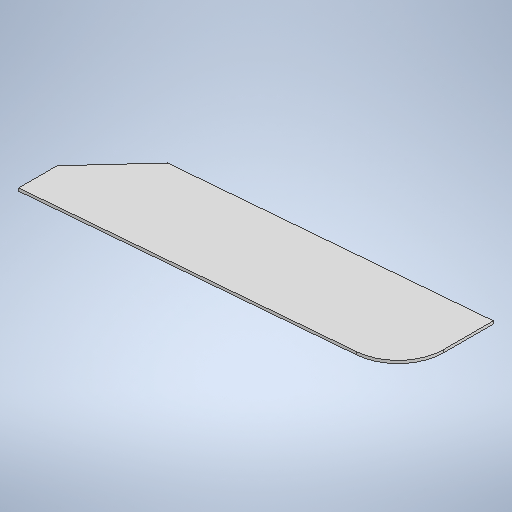
# Autodesk Inventor part: f
Saved by Autodesk Inventor 2025.2 (Build 292293000, 293)
## iProperties
Created: 2026-02-05
Part Number: f
Material: Generic
Document SubType Name: Modeling
Designer: Joefi
Density: 1 g/cm^3
Appearance: Default
Author: Joefi
Autodesk Inventor part; units mm, degrees
ref_plane "YZ Plane" through (0, 0, 0) normal (1, 0, 0) x (0, 1, 0)
ref_plane "XZ Plane" through (0, 0, 0) normal (0, 1, 0) x (-1, 0, 0)
ref_plane "XY Plane" through (0, 0, 0) normal (0, 0, 1) x (1, 0, 0)
sketch "Sketch1" plane through (0, 0, 0) normal (0, 1, 0) x (-1, 0, 0)
  line L0 (49.034, 47.4336) -> (49.034, 46.8346)
  arc A0 (47.7204, 43.4566) -> (49.034, 46.8346) centre (44.034, 46.8346) ccw
  line L1 (47.7204, 43.4566) -> (36.3172, 31.0122)
  arc A1 (33.0666, 29.4092) -> (36.3172, 31.0122) centre (32.6308, 34.3902) ccw
  line L2 (33.0666, 29.4092) -> (-42.1497, 22.8286)
  arc A2 (-47.5855, 27.8096) -> (-42.1497, 22.8286) centre (-42.5855, 27.8096) ccw
  line L3 (-47.5855, 27.8096) -> (-47.5855, 34.3574)
  arc A3 (-37.5442, 45.3156) -> (-47.5855, 34.3574) centre (-36.5855, 34.3574) ccw
  line L4 (-37.5442, 45.3156) -> (43.5982, 52.4146)
  arc A4 (49.034, 47.4336) -> (43.5982, 52.4146) centre (44.034, 47.4336) ccw
  line L5 (35.9527, 27.654) -> (51.034, 44.1124)
  line L6 (51.034, 44.1124) -> (51.034, 55.0728)
  line L7 (51.034, 55.0728) -> (-37.7185, 47.308)
  arc A5 (-37.7185, 47.308) -> (-49.5855, 34.3574) centre (-36.5855, 34.3574) ccw
  line L8 (-49.5855, 34.3574) -> (-49.5855, 20.1704)
  line L9 (-49.5855, 20.1704) -> (35.9527, 27.654)
  line L10 (35.8578, 27.8465) -> (50.834, 44.1902)
  line L11 (50.834, 44.1902) -> (50.834, 54.8545)
  line L12 (50.834, 54.8545) -> (-37.7011, 47.1087)
  arc A6 (-37.7011, 47.1087) -> (-49.3855, 34.3574) centre (-36.5855, 34.3574) ccw
  line L13 (-49.3855, 34.3574) -> (-49.3855, 20.3887)
  line L14 (-49.3855, 20.3887) -> (35.8578, 27.8465)
  dimension "d0" = 0.2
  constraints: 30 end point, 14 point on circle, 7 centre point, 5 other
  measures "d0" distance between parallel lines of L9 L14
extrude "Extrusion1" add sketch "Sketch1" along normal blind 0.8 contours L0 A0 L1 A1 L2 A2 L3 A3 L4 A4 | L9 L8 A5 L7 L6 L5 | L14 L13 A6 L12 L11 L10
body "Solid1"
